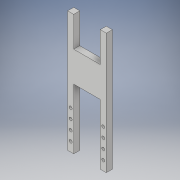
# Autodesk Inventor part: Bridge
Saved by Autodesk Inventor 2019 (Build 230136000, 136)
## iProperties
Created: 2022-07-25
Part Number: Bridge
Material: Generic
Document SubType Name: Modeling
Designer: zreik
Density: 1 g/cm^3
Appearance: Default
Author: zreik
Autodesk Inventor part; units mm, degrees
ref_plane "YZ Plane" through (0, 0, 0) normal (1, 0, 0) x (0, 1, 0)
ref_plane "XZ Plane" through (0, 0, 0) normal (0, 1, 0) x (-1, 0, 0)
ref_plane "XY Plane" through (0, 0, 0) normal (0, 0, 1) x (1, 0, 0)
sketch "Sketch1" plane through (0, 0, 0) normal (0, 0, 1) x (1, 0, 0)
  line L0 (11, 50) -> (11, 0)
  line L1 (11, 0) -> (16, 0)
  line L2 (16, 0) -> (16, 2.88)
  line L3 (11, 50) -> (0, 50)
  line L4 (0, 50) -> (0, 100) construction
  line L5 (11, 100) -> (16, 100)
  line L6 (16, 100) -> (16, 2.88)
  circle A0 centre (13.5, 7.75) radius 1.25
  circle A1 centre (13.5, 15.75) radius 1.25
  circle A2 centre (13.5, 23.75) radius 1.25
  circle A3 centre (13.5, 31.75) radius 1.25
  line L7 (-11, 50) -> (-11, 0)
  line L8 (-11, 0) -> (-16, 0)
  line L9 (-11, 50) -> (0, 50)
  line L10 (-11, 100) -> (-16, 100)
  line L11 (-16, 100) -> (-16, 2.88)
  circle A4 centre (-13.5, 7.75) radius 1.25
  circle A5 centre (-13.5, 15.75) radius 1.25
  circle A6 centre (-13.5, 23.75) radius 1.25
  circle A7 centre (-13.5, 31.75) radius 1.25
  line L12 (-16, 2.88) -> (-16, 0)
  line L13 (-11, 100) -> (-11, 75)
  line L14 (-11, 75) -> (11, 75)
  line L15 (11, 75) -> (11, 100)
  point P0 (0, 0)
  dimension "d0" = 5
  dimension "d1" = 100
  dimension "d2" = 11
  dimension "d3" = 50
  dimension "d4" = 0
  dimension "d5" = 0
  dimension "d6" = 2.5
  dimension "d7" = 2.5
  dimension "d8" = 7.75
  dimension "d9" = 0
  dimension "d10" = 8
  dimension "d11" = 2.5
  dimension "d12" = 0
  dimension "d13" = 8
  dimension "d14" = 2.5
  dimension "d15" = 2.5
  dimension "d16" = 0
  dimension "d17" = 8
  dimension "d18" = 5
  dimension "d19" = 5
  dimension "d20" = 25
  dimension "d21" = 0
  constraints: 32 end point, 9 symmetric about line, 8 centre point, 5 perpendicular, 2 parallel, 2 vertical, 1 horizontal, 4 other
  measures "d0" distance of L0.end L1.end
  measures "d1" distance between parallel lines of L1 L5
  measures "d2" distance of L0.start L3.end
  measures "d3" distance of L0.start L0.end
  measures "d4" distance from line of point (0, 0) L1
  measures "d5" distance from line of point (0, 0) L4
  measures "d6" diameter of A0
  measures "d7" distance from line of L0 A0.centre
  measures "d8" distance from line of L1 A0.centre
  measures "d9" horizontal distance of A0.centre A1.centre
  measures "d10" distance of A0.centre A1.centre
  measures "d11" diameter of A1
  measures "d12" horizontal distance of A1.centre A2.centre
  measures "d13" distance of A1.centre A2.centre
  measures "d14" diameter of A2
  measures "d15" diameter of A3
  measures "d16" horizontal distance of A2.centre A3.centre
  measures "d17" distance of A2.centre A3.centre
  measures "d18" distance between parallel lines of L6 L15
  measures "d19" distance between parallel lines of L11 L13
  measures "d20" distance between parallel lines of L5 L14
  measures "d21" vertical distance of L10.end L10.start
extrude "Extrusion1" add sketch "Sketch1" along normal blind 5
equation "\"d11\" = d6"
equation "\"d14\" = d6"
equation "\"d15\" = d6"
body "Solid1"
